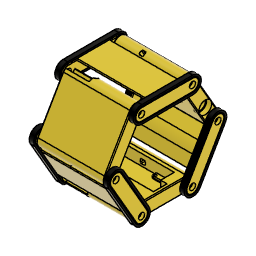
Fred (Autodesk Fusion 360 design; units mm, degrees)
Autodesk Fusion 360 part; units mm, degrees
note: some values were not read from the file. Chosen so that the rebuilt part matches the saved one: which bodies a step acts on. Set by a fixed rule: which sketch regions a step uses.
sketch "Sketch1" plane through (0, 0, 0) normal (1, 0, 0) x (0, 1, 0)
  line L0 (-30, 0) -> (30, 0) construction
  line L1 (-30, 8) -> (30, 8)
  line L2 (-30, -8) -> (30, -8)
  arc A0 (-30, 8) -> (-30, -8) centre (-30, 0) ccw
  arc A1 (30, -8) -> (30, 8) centre (30, 0) ccw
  dimension "d2" = 60
  dimension "d3" = 16
  constraint horizontal L0
  constraint midpoint origin L0
  constraint coincident L0.start A0.centre
  constraint coincident L0.end A1.centre
  constraint equal A0 A1
  constraint tangent L1 A1
  constraint tangent L2 A1
  constraint tangent L1 A0
  constraint tangent L2 A0
  measures "d2" distance of L0.start L0.end
  measures "d3" diameter of A0
extrude "Extrude1" add sketch "Sketch1" along normal mid plane 80 makes body 1
ref_plane "WorkPlane1" through (-35, 0, 0) normal (-1, 0, 0) x (0, -1, 0)
sketch "Sketch2" plane through (-35, 0, 0) normal (-1, 0, 0) x (0, -1, 0)
  arc A0 (30, -8) -> (30, 8) centre (30, 0) ccw
  line L0 (23.8, 3) -> (24.5741, 3)
  line L1 (23.8, -3) -> (24.5741, -3)
  arc A1 (24.5741, -3) -> (24.5741, 3) centre (30, 0) ccw
  arc A2 (23.8, 3) -> (23.8, -3) centre (23.8, 0) ccw
  line L2 (35.0557, 6.2) -> (8, 6.2)
  line L3 (8, 6.2) -> (8, -6.2)
  line L4 (8, -6.2) -> (35.0557, -6.2)
  line L5 (13, 6.2) -> (13, -6.2)
  line L6 (8, 0) -> (13, 0) construction
  circle A3 centre (10.5, 0) radius 2.5
  circle A4 centre (10.5, 0) radius 1
  circle A5 centre (-30, 0) radius 1.3
  arc A6 (-30, 8) -> (-30, -8) centre (-30, 0) ccw
  dimension "d8" = 12.4
  dimension "d9" = 6
  dimension "d10" = 5
  dimension "d11" = 17
  dimension "d12" = 2
  dimension "d30" = 2.6
  constraint concentric A0 A1
  constraint coincident A2.centre A1
  constraint horizontal A0.centre A2.centre
  constraint tangent L0 A2
  constraint tangent L1 A2
  constraint horizontal L0.start L0.end
  constraint horizontal L1
  constraint coincident A0 L2.start
  constraint horizontal L2
  constraint perpendicular L2 L3
  constraint coincident A0 L4.end
  constraint perpendicular L3 L4
  constraint tangent A1 L2
  constraint tangent A1 L4
  constraint coincident L2 L5.start
  constraint coincident L4 L5.end
  constraint perpendicular L4 L5
  constraint midpoint L3 L6.start
  constraint midpoint L5 L6.end
  constraint midpoint L6 A3.centre
  constraint coincident L6.end A3
  constraint concentric A3 A4
  constraint concentric A5 A6
  measures "d8" diameter of A1
  measures "d9" diameter of A2
  measures "d10" distance of L3 L5
  measures "d11" distance of A0.centre L5
  measures "d12" diameter of A4
  measures "d30" diameter of A5
extrude "Extrude2" cut sketch "Sketch2" along normal up to surface (5 mm away) contours A0 A1 L2 L4 | L0 L1 A1 A2 | A3 | A4 | A5 bodies 1
extrude "Extrude3" cut sketch "Sketch2" against normal blind 5 contours L3 L4 L5 A3 | L2 L3 L5 A3 | A3 | A5 bodies 1
extrude "Extrude4" cut sketch "Sketch2" against normal blind 23.5 contours A0 A1 L2 L4 | L0 L1 A1 A2 L2 L4 L5 | L0 L1 A1 A2 bodies 1
extrude "Extrude5" cut sketch "Sketch2" against normal blind 13 contours A4 bodies 1
sketch "Sketch3" plane through (-11.5, 0, 0) normal (-1, 0, 0) x (0, -1, 0)
  line L0 (13, 6.2) -> (13, -6.2)
  line L1 (13, -6.2) -> (35.0557, -6.2)
  arc A0 (35.0557, -6.2) -> (35.0557, 6.2) centre (30, 0) ccw
  line L2 (35.0557, 6.2) -> (13, 6.2)
  arc A1 (30, -8) -> (30, 8) centre (30, 0) ccw
  arc A2 (-30, 8) -> (-30, -8) centre (-30, 0) ccw
  line L3 (-37.5993, 2.5) -> (37.5993, 2.5)
  line L4 (37.5993, -2.5) -> (-37.5993, -2.5)
  dimension "d22" = 2.5
  dimension "d23" = 2.5
  constraint coincident A2 L3.start
  constraint coincident A1 L3.end
  constraint coincident A0 L3.end
  constraint coincident A1 L4.start
  constraint coincident A2 L4.end
  constraint parallel L1 L4
  constraint horizontal L3
  measures "d22" distance of A0.centre L3
  measures "d23" distance of A0.centre L4
extrude "Extrude6" cut sketch "Sketch3" against normal blind 2 contours L0 A0 A1 L3 L4 | L0 A2 L3 L4 bodies 1
sketch "Sketch5" plane through (40, 0, 0) normal (1, 0, 0) x (0, 1, 0)
  arc A0 (-30, 8) -> (-30, -8) centre (-30, 0) ccw
  line L0 (-30, -8) -> (30, -8)
  arc A1 (30, -8) -> (30, 8) centre (30, 0) ccw
  line L1 (30, 8) -> (-30, 8)
  circle A2 centre (-30, 0) radius 1.3
  circle A3 centre (30, 0) radius 1.3
  circle A4 centre (30, 0) radius 1.3
  constraint equal A2 A3
  constraint equal A3 A4
  constraint concentric A1 A3
  constraint concentric A0 A2
extrude "Extrude7" cut sketch "Sketch5" against normal blind 10 contours A2 | A3 A4 bodies 1
fillet "Fillet1" radius 1 12 edges at (-40, -32.6833, 7.5366) (-40, 0, 8) (-40, 38, 0) (-40, 0, -8) (-40, -32.6833, -7.5366) (40, 0, -8) (40, 38, 0) (40, 0, 8) (40, -38, 0) (-40, 31.212, 0.4701) (40, -31.212, 0.4701) (40, 28.788, 0.4701) on bodies 1
fillet "Fillet1" radius 0.5 4 edges at (-25.75, -35.0557, 6.2) (-25.75, -35.0557, -6.2) (-30, -9.5677, -0.3616) (-30, -13, 0) on bodies 1
ref_plane "WorkPlane2" through (-40.2, 1.8752, 0) normal (-1, 0, 0) x (0, -1, 0)
sketch "Sketch6" plane through (-40.2, 0, 0) normal (-1, 0, 0) x (0, -1, 0)
  arc A0 (37.5993, 2.5) -> (33.5952, 7.1467) centre (30, 0) ccw
  line L0 (30, 0) -> (60, 51.9615) construction
  line L1 (30, 0) -> (90, 0) construction
  line L2 (36.9282, -4) -> (66.9282, 47.9615)
  line L3 (23.0718, 4) -> (53.0718, 55.9615)
  arc A1 (23.0718, 4) -> (36.9282, -4) centre (30, 0) ccw
  arc A2 (66.9282, 47.9615) -> (53.0718, 55.9615) centre (60, 51.9615) ccw
  circle A3 centre (60, 51.9615) radius 1.5
  circle A4 centre (60, 51.9615) radius 3.6
  circle A5 centre (30, 0) radius 1.5
  circle A6 centre (30, 0) radius 3.6
  line L4 (36.3617, 15.2007) -> (27.063, 2.0818)
  line L5 (39.9833, 13.1098) -> (33.2714, -1.5027)
  arc A7 (39.9833, 13.1098) -> (36.3617, 15.2007) centre (38.075, 13.9863) ccw
  line L6 (38.0718, 29.9808) -> (51.9282, 21.9808) construction
  circle A8 centre (30, 0) radius 8 construction
  line L7 (37.9645, -0.7527) -> (53.2383, 56.25) construction
  line L8 (41.9282, 4.6603) -> (41.0622, 5.1603)
  line L9 (41.0622, 5.1603) -> (46.4212, 25.1603)
  line L10 (61.0622, 39.8013) -> (46.4212, 25.1603)
  line L11 (61.9282, 39.3013) -> (61.0622, 39.8013)
  dimension "d35" = 60
  dimension "d36" = 60
  dimension "d37" = 3
  dimension "d38" = 7.2
  dimension "d39" = 4.2
  dimension "d40" = 16.15
  dimension "d41" = 15
  dimension "d42" = 20
  dimension "d43" = 1
  constraint concentric A0 A1
  constraint equal A0 A1
  constraint horizontal L1
  constraint coincident A0.centre L0.start
  constraint coincident L0.end A2.centre
  constraint equal A1 A2
  constraint tangent L2 A2
  constraint tangent L3 A2
  constraint tangent L3 A1
  constraint tangent L2 A1
  constraint concentric A2 A3
  constraint concentric A2 A4
  constraint concentric A1 A5
  constraint concentric A0 A6
  constraint equal A3 A5
  constraint equal A4 A6
  constraint coincident L0 A7.centre
  constraint coincident A6 L4.end
  constraint tangent A6 L4
  constraint coincident A6 L5.end
  constraint tangent A6 L5
  constraint tangent L4 A7
  constraint tangent L5 A7
  constraint midpoint L3 L6.start
  constraint midpoint L2 L6.end
  constraint coincident A8 L7.start
  constraint coincident L3 L7.end
  constraint coincident L2 L8.start
  constraint perpendicular L2 L8
  constraint coincident L6 L9.end
  constraint parallel L7 L9
  constraint symmetric L6 L8.start L11.start
  constraint symmetric L6 L8.end L10.start
  constraint symmetric L6 L9.end L10.end
  measures "d35" angle of L0 L1
  measures "d36" distance of A0.centre L0.end
  measures "d37" diameter of A3
  measures "d38" diameter of A4
  measures "d39" diameter of A7
  measures "d40" distance of A0.centre A7.centre
  measures "d41" angle of L2 L7
  measures "d42" distance of L6 L8
  measures "d43" distance of L8.start L8.end
extrude "Extrude8" add sketch "Sketch6" along normal blind 5.8 separate body contours L2 L3 A1 A2 L8 L9 L10 L11 | L2 L8 L9 L10 L11 | A6 L4 L5 A7 makes body 2
extrude "Extrude9" add sketch "Sketch6" along normal blind 2 contours A4 | A6 bodies 2
mirror "Mirror1" about plane through (0, 0, 0) normal (1, 0, 0) of bodies 2 makes body 3
extrude "Extrude10" add sketch "Sketch6" against normal up to surface (80.4 mm away) contours L2 L8 L9 L10 L11 bodies 2 3
extrude "Extrude11" cut sketch "Sketch6" along normal up to surface (5.8 mm away) contours A6 | A6 L4 L5 A7 bodies 2
extrude "Extrude12" add sketch "Sketch6" along normal blind 3.3 contours A6 L4 L5 A7 bodies 2
fillet "Fillet2" radius 1 20 edges at (-46, -51.9282, 21.9808) (-46, -64, 58.8897) (-46, -38.0718, 29.9808) (-46, -26, -6.9282) (-40.2, -39.4282, 0.3301) (-40.2, -26, -6.9282) (-40.2, -38.0718, 29.9808) (-40.2, -64, 58.8897) (-40.2, -64.4282, 43.6314) (40.2, -39.4282, 0.3301) (40.2, -26, -6.9282) (40.2, -38.0718, 29.9808) (40.2, -64, 58.8897) (40.2, -64.4282, 43.6314) (46, -51.9282, 21.9808) (46, -64, 58.8897) (46, -38.0718, 29.9808) (46, -26, -6.9282) (0, -61.9282, 39.3013) (0, -41.9282, 4.6603) on bodies 2 3
fillet "Fillet2" radius 0.5 4 edges at (-46, -39.125, 15.805) (-46, -36.6274, 5.8036) (-46, -28.2, -3.1177) (-46, -31.7123, 8.6412) on bodies 2 3
fillet "Fillet2" radius 25 1 edges at (0, -46.4212, 25.1603) on bodies 2 3
sketch "Sketch7" plane through (-46, 0, 0) normal (-1, 0, 0) x (0, -1, 0)
  line L0 (36.0622, -3.5) -> (66.0622, 48.4615)
  arc A0 (66.0622, 48.4615) -> (53.9378, 55.4615) centre (60, 51.9615) ccw
  line L1 (53.9378, 55.4615) -> (23.9378, 3.5)
  arc A1 (23.9378, 3.5) -> (36.0622, -3.5) centre (30, 0) ccw
  circle A2 centre (60, 51.9615) radius 3.6
  arc A3 (40.4377, 12.9011) -> (35.9538, 15.4898) centre (38.075, 13.9863) ccw
  line L2 (40.4377, 12.9011) -> (33.7258, -1.7114)
  arc A4 (26.655, 2.3709) -> (33.7258, -1.7114) centre (30, 0) ccw
  line L3 (26.655, 2.3709) -> (35.9538, 15.4898)
  arc A5 (23.0718, 4) -> (36.9282, -4) centre (30, 0) ccw
  line L4 (36.9282, -4) -> (66.9282, 47.9615)
  line L5 (53.0718, 55.9615) -> (23.0718, 4)
  arc A6 (66.9282, 47.9615) -> (53.0718, 55.9615) centre (60, 51.9615) ccw
  line L6 (38.6603, -5) -> (68.6603, 46.9615)
  arc A7 (68.6603, 46.9615) -> (51.3397, 56.9615) centre (60, 51.9615) ccw
  line L7 (51.3397, 56.9615) -> (21.3397, 5)
  arc A8 (21.3397, 5) -> (38.6603, -5) centre (30, 0) ccw
  line L8 (36.0622, -3.5) -> (66.0622, 48.4615)
  arc A9 (66.0622, 48.4615) -> (53.9378, 55.4615) centre (60, 51.9615) ccw
  line L9 (53.9378, 55.4615) -> (23.9378, 3.5)
  arc A10 (23.9378, 3.5) -> (36.0622, -3.5) centre (30, 0) ccw
  dimension "d62" = 2
  dimension "d63" = -1
extrude "Extrude13" add sketch "Sketch7" along normal blind 0.25 separate body contours A5 L4 L5 A6 | L6 A7 L7 A8 makes body 4
extrude "Extrude14" add sketch "Sketch7" against normal blind 5 contours L6 A7 L7 A8 bodies 4
mirror "Mirror2" about plane through (0, 0, 0) normal (1, 0, 0) of bodies 4 makes body 5
sketch "Sketch8" plane through (0, 0, 0) normal (0, 1, 0) x (1, 0, 0)
  line L0 (0, 0) -> (30, -51.9615) construction
  line L1 (30, -51.9615) -> (-30, -51.9615) construction
  line L2 (-30, -51.9615) -> (0, 0) construction
  line L3 (41.2, -5.5263) -> (-41.2, -5.5263)
  dimension "d70" = 60
  dimension "d72" = 120
  constraint coincident L0.start L2.end
  constraint horizontal L1
  constraint equal L0 L2
  measures "d70" distance of L1.end L0.start
  measures "d72" angle of L2 L3
pattern_circular "C-Pattern1" count 3 over 360 about axis through (30, 0, 51.9615) along (-1, 0, 0) of bodies 2 4 5 1 makes body 6 at (-13, -33.0718, 82.6025) makes body 7 at (-13, 43.0718, 65.282) makes body 8 at (-13.7333, 6.3334, 111.923) makes body 9 at (13.7333, 55.0949, 27.4656) makes body 10 at (-46.25, -10, 112.923) makes body 11 at (-46.25, 57.7942, 30.141) makes body 12 at (46.25, -10, 112.923) makes body 13 at (46.25, 57.7942, 30.141)
sketch "Sketch9" plane through (0, 0, 8) normal (0, 0, 1) x (-1, 0, 0)
  line L0 (-39, 30) -> (-39, -30)
  line L1 (-39, -30) -> (39, -30)
  line L2 (39, -30) -> (39, 30)
  line L3 (39, 30) -> (-39, 30)
  line L4 (38, -26) -> (38, 6)
  line L5 (38, 6) -> (-36, 6)
  line L6 (-36, 6) -> (-36, -10)
  line L7 (-36, -10) -> (-28.5, -10)
  line L8 (-28.5, -10) -> (-28.5, -26)
  line L9 (-28.5, -26) -> (38, -26)
  line L10 (35.5, -26) -> (35.5, 6)
  circle A0 centre (-25.5, -23) radius 1.35
  circle A1 centre (-9.5, -23) radius 1.35
  line L11 (-6.5, -23) -> (-6.5, -26)
  line L12 (-9.5, -20) -> (-28.5, -20)
  arc A2 (-6.5, -23) -> (-9.5, -20) centre (-9.5, -23) ccw
  line L13 (40, 30) -> (40, -30)
  dimension "d75" = 32
  dimension "d76" = 66.5
  dimension "d78" = 4
  dimension "d79" = 16
  dimension "d80" = 2.5
  dimension "d81" = 2.7
  dimension "d82" = 3
  dimension "d83" = 16
  dimension "d84" = 3
  dimension "d97" = 74
  dimension "d143" = 2
  constraint parallel L2 L4
  constraint perpendicular L4 L5
  constraint perpendicular L5 L6
  constraint perpendicular L6 L7
  constraint perpendicular L7 L8
  constraint horizontal L9
  constraint coincident L9 L10.start
  constraint coincident L5 L10.end
  constraint perpendicular L5 L10
  constraint equal A0 A1
  constraint horizontal A0.centre A1.centre
  constraint concentric A1 A2
  constraint tangent L9 A2
  constraint coincident L9 L11.end
  constraint tangent L11 A2
  constraint coincident L8 L12.end
  constraint perpendicular L8 L12
  constraint vertical L11
  constraint tangent L12 A2
  measures "d75" distance of L4.start L4.end
  measures "d76" distance of L4.start L8.end
  measures "d78" distance of L1 L9
  measures "d79" distance of L5.end L6.end
  measures "d80" distance of L4 L10
  measures "d81" diameter of A0
  measures "d82" distance of L8 A0.centre
  measures "d83" distance of A0.centre A1.centre
  measures "d84" distance of L9 A1.centre
  measures "d97" distance of L4.end L5.end
  measures "d143" distance of L4 L13
extrude "Extrude15" cut sketch "Sketch9" against normal blind 13 contours L5 L6 L7 L8 L9 L10 L11 L12 A2 bodies 1
extrude "Extrude16" cut sketch "Sketch9" against normal blind 11 contours L4 L5 L9 L10 | L8 L9 L11 L12 A2 bodies 1
extrude "Extrude17" cut sketch "Sketch9" against normal blind 15.6 contours A0 | A1 bodies 1
sketch "Sketch10" plane through (-38, 0, 0) normal (1, 0, 0) x (0, 1, 0)
  line L0 (-6, 8) -> (-6, -3)
  line L1 (-6, -3) -> (26, -3)
  line L2 (26, -3) -> (26, 8)
  line L3 (11.5, 5) -> (3.5, 5)
  line L4 (3.5, 5) -> (3.5, 2)
  line L5 (3.5, 2) -> (11.5, 2)
  line L6 (11.5, 2) -> (11.5, 5)
  line L7 (26, 8) -> (-6, 8)
  dimension "d91" = 8
  dimension "d92" = 9.5
  dimension "d93" = 3
  dimension "d94" = 5
  constraint horizontal L3
  constraint vertical L4
  constraint horizontal L5
  constraint vertical L6
  measures "d91" distance of L3.start L3.end
  measures "d92" distance of L0 L4
  measures "d93" distance of L3.start L5.end
  measures "d94" distance of L1 L5
extrude "Extrude18" cut sketch "Sketch10" against normal up to surface (2 mm away) contours L3 L4 L5 L6 bodies 1
extrude "Extrude29" cut 1 faces at (-9.5, 29.9946, 0.1694) along direction (1, 0, 0) blind 4 on bodies 1 bodies 1
fillet "Fillet4" radius 1 14 edges at (-39, 11.5, 2) (-39, 3.5, 2) (19, 20, -3) (7.3787, 20.8787, -3) (6.5, 24.5, -3) (-35.5, 10, -3) (-9.5, -21.7997, -2.5) (-9.5, -21.7997, 2.5) (-11.5, -9.5, -2.5) (-11.5, -9.5, 2.5) (-5.5, 31.7997, 2.5) (-5.5, 31.7997, -2.5) (-11.5, 31.7997, -2.5) (-11.5, 31.7997, 2.5) on bodies 1
sketch "Sketch11" plane through (0, -60.5718, 34.9711) normal (0, 0.866025, -0.5) x (-1, 0, 0)
  line L0 (-39, 75) -> (-39, 15)
  line L1 (-39, 15) -> (39, 15)
  line L2 (39, 15) -> (39, 75)
  line L3 (39, 75) -> (-39, 75)
  line L4 (-31, 19) -> (31, 19)
  line L5 (31, 19) -> (31, 35)
  line L6 (31, 35) -> (37, 35)
  line L7 (37, 35) -> (37, 51)
  line L8 (37, 51) -> (-37, 51)
  line L9 (-37, 51) -> (-37, 35)
  line L10 (-37, 35) -> (-31, 35)
  line L11 (-31, 35) -> (-31, 19)
  line L12 (0, 51) -> (0, 75) construction
  line L13 (0, 51) -> (0, 19) construction
  dimension "d101" = 62
  dimension "d102" = 74
  dimension "d103" = 4
  dimension "d104" = 16
  dimension "d105" = 16
  constraint parallel L1 L4
  constraint perpendicular L1 L5
  constraint perpendicular L5 L6
  constraint perpendicular L1 L7
  constraint perpendicular L7 L8
  constraint perpendicular L8 L9
  constraint perpendicular L9 L10
  constraint perpendicular L10 L11
  constraint midpoint L8 L12.start
  constraint midpoint L3 L12.end
  constraint midpoint L4 L13.end
  constraint vertical L12
  constraint vertical L13
  constraint collinear L6 L10
  measures "d101" distance of L4.start L4.end
  measures "d102" distance of L7.end L8.end
  measures "d103" distance of L1 L4
  measures "d104" distance of L4.end L5.end
  measures "d105" distance of L6.end L7.end
extrude "Extrude19" cut sketch "Sketch11" against normal blind 13 contours L4 L5 L6 L7 L8 L9 L10 L11 bodies 6
sketch "Sketch12" plane through (0, 9.5, 16.4545) normal (0, 0.5, 0.866025) x (-1, 0, 0)
  line L0 (-31, 69.9423) -> (31, 69.9423)
  line L1 (31, 69.9423) -> (31, 82.9423)
  line L2 (31, 82.9423) -> (-31, 82.9423)
  line L3 (-31, 82.9423) -> (-31, 69.9423)
  line L4 (-31, 69.9423) -> (-31, 72.9423)
  line L5 (-31, 69.9423) -> (-28, 69.9423)
  line L6 (31, 69.9423) -> (31, 72.9423)
  line L7 (31, 69.9423) -> (28, 69.9423)
  arc A0 (-31, 72.9423) -> (-28, 69.9423) centre (-28, 72.9423) ccw
  arc A1 (28, 69.9423) -> (31, 72.9423) centre (28, 72.9423) ccw
  dimension "d108" = 3
  dimension "d109" = 3
  dimension "d110" = 3
  dimension "d111" = 3
  constraint coincident L0.start L3.end
  constraint perpendicular L0 L4
  constraint coincident L0 L5.end
  constraint perpendicular L4 L5
  constraint coincident L0.end L1.start
  constraint perpendicular L0 L6
  constraint coincident L0 L7.end
  constraint perpendicular L6 L7
  constraint tangent L5 A0
  constraint tangent L7 A1
  measures "d108" distance of L0.start L4.end
  measures "d109" distance of L0.end L6.end
  measures "d110" radius of A0
  measures "d111" radius of A1
extrude "Extrude20" add sketch "Sketch12" along normal up to surface (16 mm away) contours L0 L3 L4 L5 A0 | L0 L1 L6 L7 A1 bodies 6
extrude "Extrude30" add 1 faces at (-9.5, -60.144, 52.0509) along direction (-1, 0, 0) blind 2 on bodies 6 bodies 6
sketch "Sketch17" plane through (0, 0, 0) normal (1, 0, 0) x (0, 1, 0)
  line L0 (-35.0718, 79.1384) -> (-46.3301, 85.6384)
  arc A0 (-38.5359, 81.1384) -> (-43.7321, 84.1384) centre (-41.134, 82.6384) ccw
  arc A1 (-35.9378, 79.6384) -> (-46.3301, 85.6384) centre (-41.134, 82.6384) ccw
  dimension "d160" = 6
  dimension "d161" = 12
  constraint coincident L0 A0.centre
  constraint concentric A0 A1
  constraint coincident L0 A0.end
  constraint coincident L0 A0.start
  constraint coincident L0 A1.start
  measures "d160" diameter of A0
  measures "d161" diameter of A1
extrude "Extrude33" cut sketch "Sketch17" along normal mid plane 6 contours L0 A0 A1 bodies 6
fillet "Fillet5" radius 1 4 edges at (-9.5, -36.2652, 98.0714) (-9.5, -31.9351, 95.5714) (-11.5, -42.4151, 87.4195) (-11.5, -38.0849, 84.9195) on bodies 6
sketch "Sketch14" plane through (0, 60.5718, 34.9711) normal (0, -0.866025, -0.5) x (1, 0, 0)
  line L0 (39, 15) -> (39, 75)
  line L1 (39, 75) -> (-39, 75)
  line L2 (-39, 75) -> (-39, 15)
  line L3 (-39, 15) -> (39, 15)
  line L4 (22, 39) -> (-22, 39)
  line L5 (-22, 39) -> (-22, 71)
  line L6 (-22, 71) -> (22, 71)
  line L7 (22, 71) -> (22, 39)
  line L8 (0, 71) -> (0, 75) construction
  circle A0 centre (15.2, 46.9) radius 1.35
  circle A1 centre (-15.2, 63.1) radius 1.35
  circle A2 centre (15.2, 46.9) radius 4
  circle A3 centre (-15.2, 63.1) radius 4
  dimension "d118" = 4
  dimension "d119" = 44
  dimension "d120" = 32
  dimension "d121" = 2.7
  dimension "d123" = 8
  dimension "d124" = 6.8
  dimension "d125" = 24.1
  dimension "d126" = 6.8
  dimension "d127" = 7.9
  constraint horizontal L4
  constraint vertical L5
  constraint horizontal L6
  constraint vertical L7
  constraint midpoint L6 L8.start
  constraint midpoint L1 L8.end
  constraint vertical L8
  constraint equal A0 A1
  constraint concentric A0 A2
  constraint concentric A1 A3
  constraint equal A2 A3
  measures "d118" distance of L1 L6
  measures "d119" distance of L5.end L6.end
  measures "d120" distance of L4.end L5.end
  measures "d121" diameter of A0
  measures "d123" diameter of A2
  measures "d124" distance of L7 A0.centre
  measures "d125" distance of L6 A0.centre
  measures "d126" distance of L5 A1.centre
  measures "d127" distance of L6 A1.centre
extrude "Extrude23" cut sketch "Sketch14" against normal blind 15.6 contours A0 | A1 bodies 7
extrude "Extrude24" cut sketch "Sketch14" against normal blind 14 contours L4 L5 L6 L7 bodies 7
extrude "Extrude25" cut sketch "Sketch14" against normal blind 12 contours A2 | A3 bodies 7
sketch "Sketch15" plane through (0, 0, 0) normal (1, 0, 0) x (0, 1, 0)
  circle A0 centre (51.05, 67.4634) radius 6.1
  line L0 (23.0718, 99.923) -> (53.0718, 47.9615)
  line L1 (41.0718, 68.7461) -> (53.1962, 75.7461)
  line L2 (53.1962, 75.7461) -> (55.6962, 71.416)
  line L3 (45.7672, 64.4134) -> (42.7172, 69.6961)
  dimension "d134" = 12.2
  dimension "d135" = 8
  constraint tangent A0 L1
  constraint coincident L1.end L2.start
  constraint coincident A0 L2.end
  constraint perpendicular L1 L2
  constraint coincident A0 L3.start
  constraint coincident L1 L3.end
  constraint tangent A0 L3
  constraint perpendicular L1 L3
  measures "d134" diameter of A0
  measures "d135" distance of A0.centre L0
extrude "Extrude26" cut sketch "Sketch15" along normal up to surface (22 mm away) contours A0 L1 L2 | A0 L1 L3 bodies 7
extrude "Extrude27" cut sketch "Sketch15" along normal up to surface (40 mm away) contours A0 bodies 7
sketch "Sketch16" plane through (40, 0, 0) normal (1, 0, 0) x (0, 1, 0)
  circle A0 centre (51.05, 67.4634) radius 6.1
  circle A1 centre (60, 51.9615) radius 2.3
  line L0 (66.0622, 55.4615) -> (36.0622, 107.423)
  arc A2 (36.0622, 107.423) -> (23.9378, 100.423) centre (30, 103.923) ccw
  line L1 (23.9378, 100.423) -> (53.9378, 48.4615)
  arc A3 (53.9378, 48.4615) -> (66.0622, 55.4615) centre (60, 51.9615) ccw
  circle A4 centre (30, 103.923) radius 2.3
  circle A5 centre (51.05, 67.4634) radius 7.5
  dimension "d140" = 15
  constraint concentric A0 A5
  measures "d140" diameter of A5
extrude "Extrude28" cut sketch "Sketch16" against normal blind 6 contours L0 L1 A5 | L0 A5 | L1 A5 bodies 7
extrude "Extrude32" cut 2 faces at (-9.5, 57.8114, 54.0856) (-9.5, 29.856, 103.8337) along direction (1, 0, 0) blind 3 on bodies 7 bodies 7
fillet "Fillet6" radius 1 10 edges at (-6.5, 26.9351, 104.2316) (-6.5, 31.2652, 106.7316) (-11.5, 31.2652, 106.7316) (-11.5, 26.9351, 104.2316) (-6.5, 53.7348, 57.8132) (-6.5, 58.0649, 60.3132) (-11.5, 51.9151, 70.965) (-11.5, 47.5849, 68.465) (11.4707, 46.7909, 82.8404) (-18.9293, 38.6909, 96.87) on bodies 7
equation "length = 60 mm" comment "pivot to pivot length"
equation "d2 = length"
equation "d36 = length"
equation "d70 = length"
